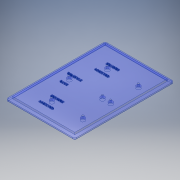
# Autodesk Inventor part: top
Saved by Autodesk Inventor 2017 SP1 (Build 210196100, 196)
## iProperties
Created: 2016-12-24
Part Number: top
Material: Generic
Document SubType Name: Modeling
Designer: wsh32
Density: 1 g/cm^3
Appearance: Clear - Blue
Author: wsh32
Autodesk Inventor part; units mm, degrees
(part 1 of 2)
ref_plane "YZ Plane" through (0, 0, 0) normal (1, 0, 0) x (0, 1, 0)
ref_plane "XZ Plane" through (0, 0, 0) normal (0, 1, 0) x (-1, 0, 0)
ref_plane "XY Plane" through (0, 0, 0) normal (0, 0, 1) x (1, 0, 0)
sketch "Sketch1" plane through (0, 0, 0) normal (0, 1, 0) x (-1, 0, 0)
  line L0 (0, 0) -> (-106.68, 0)
  line L1 (-106.68, 0) -> (-106.68, -153.67)
  line L2 (-106.68, -153.67) -> (0, -153.67)
  line L3 (0, -153.67) -> (0, 0)
  dimension "d0" = 153.67
  dimension "d1" = 106.68
  constraints: 8 end point, 2 parallel, 1 horizontal, 1 perpendicular
  measures "d0" distance of L2.end L0.start
  measures "d1" distance of L1.end L2.end
extrude "Extrusion1" add sketch "Sketch1" along normal blind 3.175
sketch "Sketch2" plane through (0, 3.175, 0) normal (0, 1, 0) x (1, 0, 0)
  line L0 (0, 0) -> (106.68, 0) projected
  line L1 (106.68, 0) -> (106.68, 153.67) projected
  line L2 (106.68, 153.67) -> (0, 153.67) projected
  line L3 (0, 153.67) -> (0, 0) projected
  line L4 (5.08, 5.08) -> (101.6, 5.08)
  line L5 (101.6, 5.08) -> (101.6, 148.59)
  line L6 (101.6, 148.59) -> (5.08, 148.59)
  line L7 (5.08, 148.59) -> (5.08, 5.08)
  dimension "d4" = 5.08
  constraints: 8 end point, 3 other
  measures "d4" distance between parallel lines of L3 L7
extrude "Extrusion2" add sketch "Sketch2" along normal blind 3.175 contours L7 L6 L5 L4
sketch "Sketch3" plane through (0, 0, 0) normal (0, -1, 0) x (1, 0, 0)
  line L0 (5.08, -5.08) -> (101.6, -5.08) construction
  line L1 (101.6, -5.08) -> (101.6, -148.59) construction
  line L2 (101.6, -148.59) -> (5.08, -148.59) construction
  line L3 (5.08, -148.59) -> (5.08, -5.08) construction
  line L4 (37.2533, -33.782) -> (85.5133, -33.782) construction
  line L5 (85.5133, -33.782) -> (85.5133, -119.888) construction
  line L6 (85.5133, -119.888) -> (37.2533, -119.888) construction
  line L7 (37.2533, -119.888) -> (37.2533, -33.782) construction
  line L8 (37.2533, -76.835) -> (85.5133, -76.835) construction
  point P0 (0, 0)
  point P1 (21.1667, -76.835)
  dimension "d7" = 28.702
  dimension "d8" = 28.702
  dimension "d9" = 16.0867
  dimension "d10" = 16.0867
  dimension "d11" = 16.0867
  dimension "d12" = 48.26
  dimension "d13" = 86.106
  constraints: 10 end point, 4 coincident, 2 midpoint, 2 parallel, 1 horizontal, 1 perpendicular, 1 point on line
  measures "d7" distance between parallel lines of L0 L4
  measures "d8" distance between parallel lines of L2 L6
  measures "d9" distance from line of L3 point (21.167, -76.835)
  measures "d10" distance from line of L7 point (21.167, -76.835)
  measures "d11" distance between parallel lines of L1 L5
  measures "d12" distance of L4.start L4.end
  measures "d13" distance of L4.end L5.end
hole "Hole1" at (37.2533, 0, -33.782) at (85.5133, 0, -33.782) at (21.1667, 0, -76.835) at (37.2533, 0, -119.888) at (85.5133, 0, -119.888) direction (0, 1, 0) diameter 3.175 end through all counterbore diameter 6.35 counterbore depth 3.175
sketch "Sketch4" plane through (0, 0, 0) normal (0, -1, 0) x (1, 0, 0)
  line L0 (31.5383, -22.987) -> (42.9683, -22.987) construction
  line L1 (42.9683, -22.987) -> (42.9683, -28.067) construction
  line L2 (42.9683, -28.067) -> (31.5383, -28.067) construction
  line L3 (31.5383, -28.067) -> (31.5383, -22.987) construction
  line L4 (31.5383, -39.497) -> (42.9683, -39.497) construction
  line L5 (42.9683, -39.497) -> (42.9683, -44.577) construction
  line L6 (42.9683, -44.577) -> (31.5383, -44.577) construction
  line L7 (31.5383, -44.577) -> (31.5383, -39.497) construction
  line L8 (15.4517, -66.04) -> (26.8817, -66.04) construction
  line L9 (26.8817, -66.04) -> (26.8817, -71.12) construction
  line L10 (26.8817, -71.12) -> (15.4517, -71.12) construction
  line L11 (15.4517, -71.12) -> (15.4517, -66.04) construction
  line L12 (15.4517, -82.55) -> (26.8817, -82.55) construction
  line L13 (26.8817, -82.55) -> (26.8817, -87.63) construction
  line L14 (26.8817, -87.63) -> (15.4517, -87.63) construction
  line L15 (15.4517, -87.63) -> (15.4517, -82.55) construction
  line L16 (31.5383, -109.093) -> (42.9683, -109.093) construction
  line L17 (42.9683, -109.093) -> (42.9683, -114.173) construction
  line L18 (42.9683, -114.173) -> (31.5383, -114.173) construction
  line L19 (31.5383, -114.173) -> (31.5383, -109.093) construction
  line L20 (31.5383, -125.603) -> (42.9683, -125.603) construction
  line L21 (42.9683, -125.603) -> (42.9683, -130.683) construction
  line L22 (42.9683, -130.683) -> (31.5383, -130.683) construction
  line L23 (31.5383, -130.683) -> (31.5383, -125.603) construction
  circle A0 centre (37.2533, -119.888) radius 3.175 construction
  circle A1 centre (85.5133, -33.782) radius 3.175 construction
  circle A2 centre (37.2533, -33.782) radius 3.175 construction
  circle A3 centre (21.1667, -76.835) radius 3.175 construction
  circle A4 centre (85.5133, -119.888) radius 3.175 construction
  line L24 (0, 0) -> (106.68, 0) construction
  line L25 (0, -153.67) -> (0, 0) construction
  line L26 (106.68, -153.67) -> (0, -153.67) construction
  line L27 (106.68, 0) -> (106.68, -153.67) construction
  circle A5 centre (37.2533, -119.888) radius 5.715 construction
  circle A6 centre (21.1667, -76.835) radius 5.715 construction
  circle A7 centre (37.2533, -33.782) radius 5.715 construction
  line L28 (28.5589, -24.5835) -> (27.2794, -24.5835)
  line L29 (27.2794, -24.5835) -> (27.2794, -25.159)
  line L30 (27.2794, -25.159) -> (28.4576, -25.159)
  line L31 (28.4576, -25.159) -> (28.4576, -25.7394)
  line L32 (28.4576, -25.7394) -> (27.2794, -25.7394)
  line L33 (27.2794, -25.7394) -> (27.2794, -27.051)
  line L34 (27.2794, -27.051) -> (26.5186, -27.051)
  line L35 (26.5186, -27.051) -> (26.5186, -24.003)
  line L36 (26.5186, -24.003) -> (28.5589, -24.003)
  line L37 (28.5589, -24.003) -> (28.5589, -24.5835)
  spline S0 degree 2 poles (31.7279, -25.527) (31.7279, -26.268) (30.9375, -27.1152) (30.2508, -27.1152) knots 0 0 0 1 2 2 2
  spline S1 degree 2 poles (30.2508, -27.1152) (29.5617, -27.1152) (28.7762, -26.2581) (28.7762, -25.527) knots 0 0 0 1 2 2 2
  spline S2 degree 2 poles (28.7762, -25.527) (28.7762, -24.7934) (29.5617, -23.9388) (30.2508, -23.9388) knots 0 0 0 1 2 2 2
  spline S3 degree 2 poles (30.2508, -23.9388) (30.9375, -23.9388) (31.7279, -24.7885) (31.7279, -25.527) knots 0 0 0 1 2 2 2
  spline S4 degree 2 poles (30.9375, -25.527) (30.9375, -25.2528) (30.8264, -24.87) (30.73, -24.7489) knots 0 0 0 1 2 2 2
  spline S5 degree 2 poles (30.73, -24.7489) (30.6337, -24.623) (30.3867, -24.5143) (30.2533, -24.5143) knots 0 0 0 1 2 2 2
  spline S6 degree 2 poles (30.2533, -24.5143) (30.1125, -24.5143) (29.8828, -24.6156) (29.7766, -24.744) knots 0 0 0 1 2 2 2
  spline S7 degree 2 poles (29.7766, -24.744) (29.6827, -24.8626) (29.5666, -25.2553) (29.5666, -25.527) knots 0 0 0 1 2 2 2
  spline S8 degree 2 poles (29.5666, -25.527) (29.5666, -25.8086) (29.6778, -26.1791) (29.7741, -26.3051) knots 0 0 0 1 2 2 2
  spline S9 degree 2 poles (29.7741, -26.3051) (29.8705, -26.431) (30.1199, -26.5397) (30.2533, -26.5397) knots 0 0 0 1 2 2 2
  spline S10 degree 2 poles (30.2533, -26.5397) (30.3892, -26.5397) (30.6411, -26.4236) (30.7325, -26.3001) knots 0 0 0 1 2 2 2
  spline S11 degree 2 poles (30.7325, -26.3001) (30.8313, -26.1667) (30.9375, -25.8135) (30.9375, -25.527) knots 0 0 0 1 2 2 2
  line L38 (34.9982, -27.051) -> (34.067, -27.051)
  line L39 (34.067, -27.051) -> (33.2198, -25.9321)
  line L40 (33.2198, -25.9321) -> (32.9432, -25.9321)
  line L41 (32.9432, -25.9321) -> (32.9432, -27.051)
  line L42 (32.9432, -27.051) -> (32.1824, -27.051)
  line L43 (32.1824, -27.051) -> (32.1824, -24.003)
  line L44 (32.1824, -24.003) -> (33.4075, -24.003)
  spline S12 degree 2 poles (33.4075, -24.003) (33.6619, -24.003) (34.0374, -24.0672) (34.1979, -24.166) knots 0 0 0 1 2 2 2
  spline S13 degree 2 poles (34.1979, -24.166) (34.3609, -24.2698) (34.5536, -24.5933) (34.5536, -24.8403) knots 0 0 0 1 2 2 2
  spline S14 degree 2 poles (34.5536, -24.8403) (34.5536, -25.1886) (34.2374, -25.6258) (33.9732, -25.7542) knots 0 0 0 1 2 2 2
  line L45 (33.9732, -25.7542) -> (34.9982, -27.051)
  spline S15 degree 2 poles (33.7681, -24.9367) (33.7681, -24.8206) (33.6792, -24.6551) (33.5779, -24.6106) knots 0 0 0 1 2 2 2
  spline S16 degree 2 poles (33.5779, -24.6106) (33.5063, -24.581) (33.3309, -24.5637) (33.2, -24.5637) knots 0 0 0 1 2 2 2
  line L46 (33.2, -24.5637) -> (32.9432, -24.5637)
  line L47 (32.9432, -24.5637) -> (32.9432, -25.3837)
  line L48 (32.9432, -25.3837) -> (33.163, -25.3837)
  spline S17 degree 2 poles (33.163, -25.3837) (33.3211, -25.3837) (33.5458, -25.3442) (33.6224, -25.2825) knots 0 0 0 1 2 2 2
  spline S18 degree 2 poles (33.6224, -25.2825) (33.6965, -25.2232) (33.7681, -25.0651) (33.7681, -24.9367) knots 0 0 0 1 2 2 2
  line L49 (39.1552, -24.003) -> (38.3846, -27.051)
  line L50 (38.3846, -27.051) -> (37.5448, -27.051)
  line L51 (37.5448, -27.051) -> (37.0557, -25.1664)
  line L52 (37.0557, -25.1664) -> (36.584, -27.051)
  line L53 (36.584, -27.051) -> (35.7417, -27.051)
  line L54 (35.7417, -27.051) -> (34.971, -24.003)
  line L55 (34.971, -24.003) -> (35.7664, -24.003)
  line L56 (35.7664, -24.003) -> (36.1863, -26.0432)
  line L57 (36.1863, -26.0432) -> (36.6951, -24.003)
  line L58 (36.6951, -24.003) -> (37.4559, -24.003)
  line L59 (37.4559, -24.003) -> (37.94, -26.0457)
  line L60 (37.94, -26.0457) -> (38.3797, -24.003)
  line L61 (38.3797, -24.003) -> (39.1552, -24.003)
  line L62 (39.2046, -27.051) -> (40.2346, -24.003)
  line L63 (40.2346, -24.003) -> (41.0695, -24.003)
  line L64 (41.0695, -24.003) -> (42.0995, -27.051)
  line L65 (42.0995, -27.051) -> (41.3116, -27.051)
  line L66 (41.3116, -27.051) -> (41.1214, -26.4286)
  line L67 (41.1214, -26.4286) -> (40.163, -26.4286)
  line L68 (40.163, -26.4286) -> (39.9704, -27.051)
  line L69 (39.9704, -27.051) -> (39.2046, -27.051)
  line L70 (40.9534, -25.8753) -> (40.6422, -24.8675)
  line L71 (40.6422, -24.8675) -> (40.3285, -25.8753)
  line L72 (40.3285, -25.8753) -> (40.9534, -25.8753)
  line L73 (45.2191, -27.051) -> (44.2879, -27.051)
  line L74 (44.2879, -27.051) -> (43.4407, -25.9321)
  line L75 (43.4407, -25.9321) -> (43.1641, -25.9321)
  line L76 (43.1641, -25.9321) -> (43.1641, -27.051)
  line L77 (43.1641, -27.051) -> (42.4033, -27.051)
  line L78 (42.4033, -27.051) -> (42.4033, -24.003)
  line L79 (42.4033, -24.003) -> (43.6284, -24.003)
  spline S19 degree 2 poles (43.6284, -24.003) (43.8829, -24.003) (44.2583, -24.0672) (44.4189, -24.166) knots 0 0 0 1 2 2 2
  spline S20 degree 2 poles (44.4189, -24.166) (44.5819, -24.2698) (44.7745, -24.5933) (44.7745, -24.8403) knots 0 0 0 1 2 2 2
  spline S21 degree 2 poles (44.7745, -24.8403) (44.7745, -25.1886) (44.4584, -25.6258) (44.1941, -25.7542) knots 0 0 0 1 2 2 2
  line L80 (44.1941, -25.7542) -> (45.2191, -27.051)
  spline S22 degree 2 poles (43.9891, -24.9367) (43.9891, -24.8206) (43.9001, -24.6551) (43.7989, -24.6106) knots 0 0 0 1 2 2 2
  spline S23 degree 2 poles (43.7989, -24.6106) (43.7272, -24.581) (43.5519, -24.5637) (43.421, -24.5637) knots 0 0 0 1 2 2 2
  line L81 (43.421, -24.5637) -> (43.1641, -24.5637)
  line L82 (43.1641, -24.5637) -> (43.1641, -25.3837)
  line L83 (43.1641, -25.3837) -> (43.3839, -25.3837)
  spline S24 degree 2 poles (43.3839, -25.3837) (43.542, -25.3837) (43.7668, -25.3442) (43.8433, -25.2825) knots 0 0 0 1 2 2 2
  spline S25 degree 2 poles (43.8433, -25.2825) (43.9174, -25.2232) (43.9891, -25.0651) (43.9891, -24.9367) knots 0 0 0 1 2 2 2
  spline S26 degree 2 poles (48.1659, -25.5295) (48.1659, -25.9568) (47.7929, -26.6286) (47.5088, -26.8089) knots 0 0 0 1 2 2 2
  spline S27 degree 2 poles (47.5088, -26.8089) (47.2717, -26.9621) (46.7135, -27.051) (46.3998, -27.051) knots 0 0 0 1 2 2 2
  line L84 (46.3998, -27.051) -> (45.4464, -27.051)
  line L85 (45.4464, -27.051) -> (45.4464, -24.003)
  line L86 (45.4464, -24.003) -> (46.3899, -24.003)
  spline S28 degree 2 poles (46.3899, -24.003) (46.711, -24.003) (47.2717, -24.0845) (47.5187, -24.2426) knots 0 0 0 1 2 2 2
  spline S29 degree 2 poles (47.5187, -24.2426) (47.8176, -24.4353) (48.1659, -25.0873) (48.1659, -25.5295) knots 0 0 0 1 2 2 2
  spline S30 degree 2 poles (47.3804, -25.5245) (47.3804, -25.2232) (47.1729, -24.7934) (46.9605, -24.6724) knots 0 0 0 1 2 2 2
  spline S31 degree 2 poles (46.9605, -24.6724) (46.8049, -24.5884) (46.464, -24.5711) (46.2269, -24.5711) knots 0 0 0 1 2 2 2
  line L87 (46.2269, -24.5711) -> (46.2121, -24.5711)
  line L88 (46.2121, -24.5711) -> (46.2121, -26.4804)
  line L89 (46.2121, -26.4804) -> (46.2269, -26.4804)
  spline S32 degree 2 poles (46.2269, -26.4804) (46.4838, -26.4804) (46.837, -26.4631) (46.9975, -26.3619) knots 0 0 0 1 2 2 2
  spline S33 degree 2 poles (46.9975, -26.3619) (47.1853, -26.2433) (47.3804, -25.8259) (47.3804, -25.5245) knots 0 0 0 1 2 2 2
  line L90 (30.7325, -43.561) -> (29.8013, -43.561)
  line L91 (29.8013, -43.561) -> (28.9541, -42.4421)
  line L92 (28.9541, -42.4421) -> (28.6774, -42.4421)
  line L93 (28.6774, -42.4421) -> (28.6774, -43.561)
  line L94 (28.6774, -43.561) -> (27.9167, -43.561)
  line L95 (27.9167, -43.561) -> (27.9167, -40.513)
  line L96 (27.9167, -40.513) -> (29.1418, -40.513)
  spline S34 degree 2 poles (29.1418, -40.513) (29.3962, -40.513) (29.7717, -40.5772) (29.9322, -40.676) knots 0 0 0 1 2 2 2
  spline S35 degree 2 poles (29.9322, -40.676) (30.0952, -40.7798) (30.2879, -41.1033) (30.2879, -41.3503) knots 0 0 0 1 2 2 2
  spline S36 degree 2 poles (30.2879, -41.3503) (30.2879, -41.6986) (29.9717, -42.1358) (29.7074, -42.2642) knots 0 0 0 1 2 2 2
  line L97 (29.7074, -42.2642) -> (30.7325, -43.561)
  spline S37 degree 2 poles (29.5024, -41.4467) (29.5024, -41.3306) (29.4135, -41.1651) (29.3122, -41.1206) knots 0 0 0 1 2 2 2
  spline S38 degree 2 poles (29.3122, -41.1206) (29.2406, -41.091) (29.0652, -41.0737) (28.9343, -41.0737) knots 0 0 0 1 2 2 2
  line L98 (28.9343, -41.0737) -> (28.6774, -41.0737)
  line L99 (28.6774, -41.0737) -> (28.6774, -41.8937)
  line L100 (28.6774, -41.8937) -> (28.8973, -41.8937)
  spline S39 degree 2 poles (28.8973, -41.8937) (29.0553, -41.8937) (29.2801, -41.8542) (29.3567, -41.7925) knots 0 0 0 1 2 2 2
  spline S40 degree 2 poles (29.3567, -41.7925) (29.4308, -41.7332) (29.5024, -41.5751) (29.5024, -41.4467) knots 0 0 0 1 2 2 2
  line L101 (30.9597, -43.561) -> (30.9597, -40.513)
  line L102 (30.9597, -40.513) -> (33.0197, -40.513)
  line L103 (33.0197, -40.513) -> (33.0197, -41.0935)
  line L104 (33.0197, -41.0935) -> (31.7205, -41.0935)
  line L105 (31.7205, -41.0935) -> (31.7205, -41.6294)
  line L106 (31.7205, -41.6294) -> (32.9185, -41.6294)
  line L107 (32.9185, -41.6294) -> (32.9185, -42.2099)
  line L108 (32.9185, -42.2099) -> (31.7205, -42.2099)
  line L109 (31.7205, -42.2099) -> (31.7205, -42.9805)
  line L110 (31.7205, -42.9805) -> (33.0197, -42.9805)
  line L111 (33.0197, -42.9805) -> (33.0197, -43.561)
  line L112 (33.0197, -43.561) -> (30.9597, -43.561)
  line L113 (36.0825, -40.513) -> (35.0353, -43.561)
  line L114 (35.0353, -43.561) -> (34.2374, -43.561)
  line L115 (34.2374, -43.561) -> (33.1902, -40.513)
  line L116 (33.1902, -40.513) -> (33.983, -40.513)
  line L117 (33.983, -40.513) -> (34.6475, -42.5804)
  line L118 (34.6475, -42.5804) -> (35.3094, -40.513)
  line L119 (35.3094, -40.513) -> (36.0825, -40.513)
  line L120 (36.3666, -43.561) -> (36.3666, -40.513)
  line L121 (36.3666, -40.513) -> (38.4266, -40.513)
  line L122 (38.4266, -40.513) -> (38.4266, -41.0935)
  line L123 (38.4266, -41.0935) -> (37.1274, -41.0935)
  line L124 (37.1274, -41.0935) -> (37.1274, -41.6294)
  line L125 (37.1274, -41.6294) -> (38.3253, -41.6294)
  line L126 (38.3253, -41.6294) -> (38.3253, -42.2099)
  line L127 (38.3253, -42.2099) -> (37.1274, -42.2099)
  line L128 (37.1274, -42.2099) -> (37.1274, -42.9805)
  line L129 (37.1274, -42.9805) -> (38.4266, -42.9805)
  line L130 (38.4266, -42.9805) -> (38.4266, -43.561)
  line L131 (38.4266, -43.561) -> (36.3666, -43.561)
  line L132 (41.7611, -43.561) -> (40.8299, -43.561)
  line L133 (40.8299, -43.561) -> (39.9827, -42.4421)
  line L134 (39.9827, -42.4421) -> (39.7061, -42.4421)
  line L135 (39.7061, -42.4421) -> (39.7061, -43.561)
  line L136 (39.7061, -43.561) -> (38.9453, -43.561)
  line L137 (38.9453, -43.561) -> (38.9453, -40.513)
  line L138 (38.9453, -40.513) -> (40.1704, -40.513)
  spline S41 degree 2 poles (40.1704, -40.513) (40.4248, -40.513) (40.8003, -40.5772) (40.9608, -40.676) knots 0 0 0 1 2 2 2
  spline S42 degree 2 poles (40.9608, -40.676) (41.1238, -40.7798) (41.3165, -41.1033) (41.3165, -41.3503) knots 0 0 0 1 2 2 2
  spline S43 degree 2 poles (41.3165, -41.3503) (41.3165, -41.6986) (41.0003, -42.1358) (40.7361, -42.2642) knots 0 0 0 1 2 2 2
  line L139 (40.7361, -42.2642) -> (41.7611, -43.561)
  spline S44 degree 2 poles (40.531, -41.4467) (40.531, -41.3306) (40.4421, -41.1651) (40.3409, -41.1206) knots 0 0 0 1 2 2 2
  spline S45 degree 2 poles (40.3409, -41.1206) (40.2692, -41.091) (40.0939, -41.0737) (39.9629, -41.0737) knots 0 0 0 1 2 2 2
  line L140 (39.9629, -41.0737) -> (39.7061, -41.0737)
  line L141 (39.7061, -41.0737) -> (39.7061, -41.8937)
  line L142 (39.7061, -41.8937) -> (39.9259, -41.8937)
  spline S46 degree 2 poles (39.9259, -41.8937) (40.084, -41.8937) (40.3087, -41.8542) (40.3853, -41.7925) knots 0 0 0 1 2 2 2
  spline S47 degree 2 poles (40.3853, -41.7925) (40.4594, -41.7332) (40.531, -41.5751) (40.531, -41.4467) knots 0 0 0 1 2 2 2
  spline S48 degree 2 poles (42.9294, -43.6153) (42.5787, -43.6153) (42.0501, -43.4795) (41.8229, -43.3807) knots 0 0 0 1 2 2 2
  line L143 (41.8229, -43.3807) -> (41.8229, -42.6545)
  line L144 (41.8229, -42.6545) -> (41.892, -42.6545)
  spline S49 degree 2 poles (41.892, -42.6545) (42.1217, -42.8496) (42.6725, -43.0596) (42.9319, -43.0596) knots 0 0 0 1 2 2 2
  spline S50 degree 2 poles (42.9319, -43.0596) (42.9986, -43.0596) (43.2135, -43.0299) (43.2777, -43.0003) knots 0 0 0 1 2 2 2
  spline S51 degree 2 poles (43.2777, -43.0003) (43.3567, -42.9657) (43.4679, -42.8398) (43.4679, -42.7385) knots 0 0 0 1 2 2 2
  spline S52 degree 2 poles (43.4679, -42.7385) (43.4679, -42.6224) (43.2876, -42.4791) (43.1641, -42.447) knots 0 0 0 1 2 2 2
  spline S53 degree 2 poles (43.1641, -42.447) (43.0085, -42.405) (42.6553, -42.3334) (42.4996, -42.2791) knots 0 0 0 1 2 2 2
  spline S54 degree 2 poles (42.4996, -42.2791) (42.1464, -42.1556) (41.8402, -41.7332) (41.8402, -41.417) knots 0 0 0 1 2 2 2
  spline S55 degree 2 poles (41.8402, -41.417) (41.8402, -40.9897) (42.5639, -40.4587) (43.1073, -40.4587) knots 0 0 0 1 2 2 2
  spline S56 degree 2 poles (43.1073, -40.4587) (43.379, -40.4587) (43.9174, -40.5698) (44.1299, -40.6637) knots 0 0 0 1 2 2 2
  line L145 (44.1299, -40.6637) -> (44.1299, -41.3602)
  line L146 (44.1299, -41.3602) -> (44.0632, -41.3602)
  spline S57 degree 2 poles (44.0632, -41.3602) (43.8927, -41.2145) (43.4037, -41.0144) (43.1468, -41.0144) knots 0 0 0 1 2 2 2
  spline S58 degree 2 poles (43.1468, -41.0144) (43.0455, -41.0144) (42.8874, -41.0441) (42.7985, -41.0836) knots 0 0 0 1 2 2 2
  spline S59 degree 2 poles (42.7985, -41.0836) (42.7269, -41.1157) (42.6231, -41.2441) (42.6231, -41.3232) knots 0 0 0 1 2 2 2
  spline S60 degree 2 poles (42.6231, -41.3232) (42.6231, -41.4417) (42.7886, -41.5776) (43.0258, -41.6319) knots 0 0 0 1 2 2 2
  spline S61 degree 2 poles (43.0258, -41.6319) (43.1789, -41.6665) (43.463, -41.7332) (43.626, -41.79) knots 0 0 0 1 2 2 2
  spline S62 degree 2 poles (43.626, -41.79) (43.9421, -41.9061) (44.2509, -42.2914) (44.2509, -42.6076) knots 0 0 0 1 2 2 2
  spline S63 degree 2 poles (44.2509, -42.6076) (44.2509, -43.0621) (43.5371, -43.6153) (42.9294, -43.6153) knots 0 0 0 1 2 2 2
  line L147 (44.6436, -43.561) -> (44.6436, -40.513)
  line L148 (44.6436, -40.513) -> (46.7036, -40.513)
  line L149 (46.7036, -40.513) -> (46.7036, -41.0935)
  line L150 (46.7036, -41.0935) -> (45.4044, -41.0935)
  line L151 (45.4044, -41.0935) -> (45.4044, -41.6294)
  line L152 (45.4044, -41.6294) -> (46.6023, -41.6294)
  line L153 (46.6023, -41.6294) -> (46.6023, -42.2099)
  line L154 (46.6023, -42.2099) -> (45.4044, -42.2099)
  line L155 (45.4044, -42.2099) -> (45.4044, -42.9805)
  line L156 (45.4044, -42.9805) -> (46.7036, -42.9805)
  line L157 (46.7036, -42.9805) -> (46.7036, -43.561)
  line L158 (46.7036, -43.561) -> (44.6436, -43.561)
  spline S64 degree 2 poles (16.6762, -70.1583) (16.3254, -70.1583) (15.7969, -70.0225) (15.5696, -69.9237) knots 0 0 0 1 2 2 2
  line L159 (15.5696, -69.9237) -> (15.5696, -69.1975)
  line L160 (15.5696, -69.1975) -> (15.6388, -69.1975)
  spline S65 degree 2 poles (15.6388, -69.1975) (15.8685, -69.3926) (16.4193, -69.6026) (16.6786, -69.6026) knots 0 0 0 1 2 2 2
  spline S66 degree 2 poles (16.6786, -69.6026) (16.7453, -69.6026) (16.9602, -69.5729) (17.0244, -69.5433) knots 0 0 0 1 2 2 2
  spline S67 degree 2 poles (17.0244, -69.5433) (17.1035, -69.5087) (17.2146, -69.3828) (17.2146, -69.2815) knots 0 0 0 1 2 2 2
  spline S68 degree 2 poles (17.2146, -69.2815) (17.2146, -69.1654) (17.0343, -69.0221) (16.9108, -68.99) knots 0 0 0 1 2 2 2
  spline S69 degree 2 poles (16.9108, -68.99) (16.7552, -68.948) (16.402, -68.8764) (16.2464, -68.8221) knots 0 0 0 1 2 2 2
  spline S70 degree 2 poles (16.2464, -68.8221) (15.8932, -68.6986) (15.5869, -68.2762) (15.5869, -67.96) knots 0 0 0 1 2 2 2
  spline S71 degree 2 poles (15.5869, -67.96) (15.5869, -67.5327) (16.3106, -67.0017) (16.854, -67.0017) knots 0 0 0 1 2 2 2
  spline S72 degree 2 poles (16.854, -67.0017) (17.1257, -67.0017) (17.6642, -67.1128) (17.8766, -67.2067) knots 0 0 0 1 2 2 2
  line L161 (17.8766, -67.2067) -> (17.8766, -67.9032)
  line L162 (17.8766, -67.9032) -> (17.8099, -67.9032)
  spline S73 degree 2 poles (17.8099, -67.9032) (17.6395, -67.7575) (17.1504, -67.5574) (16.8935, -67.5574) knots 0 0 0 1 2 2 2
  spline S74 degree 2 poles (16.8935, -67.5574) (16.7923, -67.5574) (16.6342, -67.5871) (16.5453, -67.6266) knots 0 0 0 1 2 2 2
  spline S75 degree 2 poles (16.5453, -67.6266) (16.4736, -67.6587) (16.3699, -67.7871) (16.3699, -67.8662) knots 0 0 0 1 2 2 2
  spline S76 degree 2 poles (16.3699, -67.8662) (16.3699, -67.9847) (16.5354, -68.1206) (16.7725, -68.1749) knots 0 0 0 1 2 2 2
  spline S77 degree 2 poles (16.7725, -68.1749) (16.9256, -68.2095) (17.2097, -68.2762) (17.3727, -68.333) knots 0 0 0 1 2 2 2
  spline S78 degree 2 poles (17.3727, -68.333) (17.6889, -68.4491) (17.9976, -68.8344) (17.9976, -69.1506) knots 0 0 0 1 2 2 2
  spline S79 degree 2 poles (17.9976, -69.1506) (17.9976, -69.6051) (17.2838, -70.1583) (16.6762, -70.1583) knots 0 0 0 1 2 2 2
  line L163 (20.9246, -67.056) -> (19.8724, -68.8319)
  line L164 (19.8724, -68.8319) -> (19.8724, -70.104)
  line L165 (19.8724, -70.104) -> (19.1067, -70.104)
  line L166 (19.1067, -70.104) -> (19.1067, -68.869)
  line L167 (19.1067, -68.869) -> (18.0372, -67.056)
  line L168 (18.0372, -67.056) -> (18.9091, -67.056)
  line L169 (18.9091, -67.056) -> (19.5043, -68.1428)
  line L170 (19.5043, -68.1428) -> (20.0799, -67.056)
  line L171 (20.0799, -67.056) -> (20.9246, -67.056)
  line L172 (23.8121, -70.104) -> (23.076, -70.104)
  line L173 (23.076, -70.104) -> (21.9003, -67.9798)
  line L174 (21.9003, -67.9798) -> (21.9003, -70.104)
  line L175 (21.9003, -70.104) -> (21.2012, -70.104)
  line L176 (21.2012, -70.104) -> (21.2012, -67.056)
  line L177 (21.2012, -67.056) -> (22.1399, -67.056)
  line L178 (22.1399, -67.056) -> (23.113, -68.8023)
  line L179 (23.113, -68.8023) -> (23.113, -67.056)
  line L180 (23.113, -67.056) -> (23.8121, -67.056)
  line L181 (23.8121, -67.056) -> (23.8121, -70.104)
  spline S80 degree 2 poles (25.7461, -70.1633) (25.0594, -70.1633) (24.2542, -69.3334) (24.2542, -68.5825) knots 0 0 0 1 2 2 2
  spline S81 degree 2 poles (24.2542, -68.5825) (24.2542, -67.8588) (25.0619, -66.9967) (25.7485, -66.9967) knots 0 0 0 1 2 2 2
  spline S82 degree 2 poles (25.7485, -66.9967) (25.9289, -66.9967) (26.2203, -67.0387) (26.3537, -67.0733) knots 0 0 0 1 2 2 2
  spline S83 degree 2 poles (26.3537, -67.0733) (26.4574, -67.1054) (26.702, -67.2116) (26.7785, -67.2511) knots 0 0 0 1 2 2 2
  line L182 (26.7785, -67.2511) -> (26.7785, -67.9773)
  line L183 (26.7785, -67.9773) -> (26.702, -67.9773)
  spline S84 degree 2 poles (26.702, -67.9773) (26.6452, -67.9279) (26.4772, -67.7896) (26.371, -67.7254) knots 0 0 0 1 2 2 2
  spline S85 degree 2 poles (26.371, -67.7254) (26.2648, -67.6587) (26.0104, -67.5673) (25.8696, -67.5673) knots 0 0 0 1 2 2 2
  spline S86 degree 2 poles (25.8696, -67.5673) (25.7041, -67.5673) (25.4299, -67.671) (25.3039, -67.8019) knots 0 0 0 1 2 2 2
  spline S87 degree 2 poles (25.3039, -67.8019) (25.1903, -67.918) (25.0446, -68.3157) (25.0446, -68.5849) knots 0 0 0 1 2 2 2
  spline S88 degree 2 poles (25.0446, -68.5849) (25.0446, -68.869) (25.1953, -69.2568) (25.3188, -69.3753) knots 0 0 0 1 2 2 2
  spline S89 degree 2 poles (25.3188, -69.3753) (25.4373, -69.4914) (25.7288, -69.5927) (25.8745, -69.5927) knots 0 0 0 1 2 2 2
  spline S90 degree 2 poles (25.8745, -69.5927) (26.0252, -69.5927) (26.2994, -69.4914) (26.3932, -69.4297) knots 0 0 0 1 2 2 2
  spline S91 degree 2 poles (26.3932, -69.4297) (26.497, -69.3679) (26.6526, -69.237) (26.7094, -69.1852) knots 0 0 0 1 2 2 2
  line L184 (26.7094, -69.1852) -> (26.7785, -69.1852)
  line L185 (26.7785, -69.1852) -> (26.7785, -69.9015)
  spline S92 degree 2 poles (26.7785, -69.9015) (26.6946, -69.941) (26.4747, -70.0398) (26.3562, -70.0744) knots 0 0 0 1 2 2 2
  spline S93 degree 2 poles (26.3562, -70.0744) (26.2129, -70.1188) (25.9634, -70.1633) (25.7461, -70.1633) knots 0 0 0 1 2 2 2
  spline S94 degree 2 poles (11.6114, -86.6683) (11.2607, -86.6683) (10.7321, -86.5325) (10.5048, -86.4337) knots 0 0 0 1 2 2 2
  line L186 (10.5048, -86.4337) -> (10.5048, -85.7075)
  line L187 (10.5048, -85.7075) -> (10.574, -85.7075)
  spline S95 degree 2 poles (10.574, -85.7075) (10.8037, -85.9026) (11.3545, -86.1126) (11.6139, -86.1126) knots 0 0 0 1 2 2 2
  spline S96 degree 2 poles (11.6139, -86.1126) (11.6806, -86.1126) (11.8955, -86.0829) (11.9597, -86.0533) knots 0 0 0 1 2 2 2
  spline S97 degree 2 poles (11.9597, -86.0533) (12.0387, -86.0187) (12.1499, -85.8928) (12.1499, -85.7915) knots 0 0 0 1 2 2 2
  spline S98 degree 2 poles (12.1499, -85.7915) (12.1499, -85.6754) (11.9696, -85.5321) (11.8461, -85.5) knots 0 0 0 1 2 2 2
  spline S99 degree 2 poles (11.8461, -85.5) (11.6904, -85.458) (11.3372, -85.3864) (11.1816, -85.3321) knots 0 0 0 1 2 2 2
  spline S100 degree 2 poles (11.1816, -85.3321) (10.8284, -85.2086) (10.5221, -84.7862) (10.5221, -84.47) knots 0 0 0 1 2 2 2
  spline S101 degree 2 poles (10.5221, -84.47) (10.5221, -84.0427) (11.2458, -83.5117) (11.7893, -83.5117) knots 0 0 0 1 2 2 2
  spline S102 degree 2 poles (11.7893, -83.5117) (12.061, -83.5117) (12.5994, -83.6228) (12.8118, -83.7167) knots 0 0 0 1 2 2 2
  line L188 (12.8118, -83.7167) -> (12.8118, -84.4132)
  line L189 (12.8118, -84.4132) -> (12.7451, -84.4132)
  spline S103 degree 2 poles (12.7451, -84.4132) (12.5747, -84.2675) (12.0857, -84.0674) (11.8288, -84.0674) knots 0 0 0 1 2 2 2
  spline S104 degree 2 poles (11.8288, -84.0674) (11.7275, -84.0674) (11.5694, -84.0971) (11.4805, -84.1366) knots 0 0 0 1 2 2 2
  spline S105 degree 2 poles (11.4805, -84.1366) (11.4089, -84.1687) (11.3051, -84.2971) (11.3051, -84.3762) knots 0 0 0 1 2 2 2
  spline S106 degree 2 poles (11.3051, -84.3762) (11.3051, -84.4947) (11.4706, -84.6306) (11.7077, -84.6849) knots 0 0 0 1 2 2 2
  spline S107 degree 2 poles (11.7077, -84.6849) (11.8609, -84.7195) (12.1449, -84.7862) (12.308, -84.843) knots 0 0 0 1 2 2 2
  spline S108 degree 2 poles (12.308, -84.843) (12.6241, -84.9591) (12.9329, -85.3444) (12.9329, -85.6606) knots 0 0 0 1 2 2 2
  spline S109 degree 2 poles (12.9329, -85.6606) (12.9329, -86.1151) (12.219, -86.6683) (11.6114, -86.6683) knots 0 0 0 1 2 2 2
  line L190 (13.3256, -86.614) -> (13.3256, -83.566)
  line L191 (13.3256, -83.566) -> (15.3856, -83.566)
  line L192 (15.3856, -83.566) -> (15.3856, -84.1465)
  line L193 (15.3856, -84.1465) -> (14.0864, -84.1465)
  line L194 (14.0864, -84.1465) -> (14.0864, -84.6824)
  line L195 (14.0864, -84.6824) -> (15.2843, -84.6824)
  line L196 (15.2843, -84.6824) -> (15.2843, -85.2629)
  line L197 (15.2843, -85.2629) -> (14.0864, -85.2629)
  line L198 (14.0864, -85.2629) -> (14.0864, -86.0335)
  line L199 (14.0864, -86.0335) -> (15.3856, -86.0335)
  line L200 (15.3856, -86.0335) -> (15.3856, -86.614)
  line L201 (15.3856, -86.614) -> (13.3256, -86.614)
  spline S110 degree 2 poles (18.2483, -84.5268) (18.2483, -84.7393) (18.1125, -85.1246) (17.9865, -85.253) knots 0 0 0 1 2 2 2
  spline S111 degree 2 poles (17.9865, -85.253) (17.91, -85.3345) (17.7222, -85.4679) (17.6111, -85.5148) knots 0 0 0 1 2 2 2
  spline S112 degree 2 poles (17.6111, -85.5148) (17.4975, -85.5618) (17.2332, -85.6161) (17.0701, -85.6161) knots 0 0 0 1 2 2 2
  line L202 (17.0701, -85.6161) -> (16.67, -85.6161)
  line L203 (16.67, -85.6161) -> (16.67, -86.614)
  line L204 (16.67, -86.614) -> (15.9043, -86.614)
  line L205 (15.9043, -86.614) -> (15.9043, -83.566)
  line L206 (15.9043, -83.566) -> (17.0874, -83.566)
  spline S113 degree 2 poles (17.0874, -83.566) (17.3493, -83.566) (17.7321, -83.6623) (17.8877, -83.7661) knots 0 0 0 1 2 2 2
  spline S114 degree 2 poles (17.8877, -83.7661) (18.0606, -83.8822) (18.2483, -84.2625) (18.2483, -84.5268) knots 0 0 0 1 2 2 2
  spline S115 degree 2 poles (17.4629, -84.5466) (17.4629, -84.4157) (17.3394, -84.2304) (17.2554, -84.1959) knots 0 0 0 1 2 2 2
  spline S116 degree 2 poles (17.2554, -84.1959) (17.1467, -84.1489) (16.9491, -84.1341) (16.7787, -84.1341) knots 0 0 0 1 2 2 2
  line L207 (16.7787, -84.1341) -> (16.67, -84.1341)
  line L208 (16.67, -84.1341) -> (16.67, -85.048)
  line L209 (16.67, -85.048) -> (16.7243, -85.048)
  spline S117 degree 2 poles (16.7243, -85.048) (16.8306, -85.048) (17.0232, -85.0431) (17.0948, -85.0307) knots 0 0 0 1 2 2 2
  spline S118 degree 2 poles (17.0948, -85.0307) (17.1566, -85.0208) (17.2924, -84.9616) (17.3295, -84.9245) knots 0 0 0 1 2 2 2
  spline S119 degree 2 poles (17.3295, -84.9245) (17.4085, -84.8504) (17.4629, -84.6849) (17.4629, -84.5466) knots 0 0 0 1 2 2 2
  line L210 (18.6584, -86.614) -> (18.6584, -83.566)
  line L211 (18.6584, -83.566) -> (20.7184, -83.566)
  line L212 (20.7184, -83.566) -> (20.7184, -84.1465)
  line L213 (20.7184, -84.1465) -> (19.4191, -84.1465)
  line L214 (19.4191, -84.1465) -> (19.4191, -84.6824)
  line L215 (19.4191, -84.6824) -> (20.6171, -84.6824)
  line L216 (20.6171, -84.6824) -> (20.6171, -85.2629)
  line L217 (20.6171, -85.2629) -> (19.4191, -85.2629)
  line L218 (19.4191, -85.2629) -> (19.4191, -86.0335)
  line L219 (19.4191, -86.0335) -> (20.7184, -86.0335)
  line L220 (20.7184, -86.0335) -> (20.7184, -86.614)
  line L221 (20.7184, -86.614) -> (18.6584, -86.614)
  line L222 (24.0529, -86.614) -> (23.1217, -86.614)
  line L223 (23.1217, -86.614) -> (22.2745, -85.4951)
  line L224 (22.2745, -85.4951) -> (21.9978, -85.4951)
  line L225 (21.9978, -85.4951) -> (21.9978, -86.614)
  line L226 (21.9978, -86.614) -> (21.2371, -86.614)
  line L227 (21.2371, -86.614) -> (21.2371, -83.566)
  line L228 (21.2371, -83.566) -> (22.4622, -83.566)
  spline S120 degree 2 poles (22.4622, -83.566) (22.7166, -83.566) (23.092, -83.6302) (23.2526, -83.729) knots 0 0 0 1 2 2 2
  spline S121 degree 2 poles (23.2526, -83.729) (23.4156, -83.8328) (23.6083, -84.1563) (23.6083, -84.4033) knots 0 0 0 1 2 2 2
  spline S122 degree 2 poles (23.6083, -84.4033) (23.6083, -84.7516) (23.2921, -85.1888) (23.0278, -85.3172) knots 0 0 0 1 2 2 2
  line L229 (23.0278, -85.3172) -> (24.0529, -86.614)
  spline S123 degree 2 poles (22.8228, -84.4997) (22.8228, -84.3836) (22.7339, -84.2181) (22.6326, -84.1736) knots 0 0 0 1 2 2 2
  spline S124 degree 2 poles (22.6326, -84.1736) (22.561, -84.144) (22.3856, -84.1267) (22.2547, -84.1267) knots 0 0 0 1 2 2 2
  line L230 (22.2547, -84.1267) -> (21.9978, -84.1267)
  line L231 (21.9978, -84.1267) -> (21.9978, -84.9467)
  line L232 (21.9978, -84.9467) -> (22.2177, -84.9467)
  spline S125 degree 2 poles (22.2177, -84.9467) (22.3757, -84.9467) (22.6005, -84.9072) (22.6771, -84.8455) knots 0 0 0 1 2 2 2
  spline S126 degree 2 poles (22.6771, -84.8455) (22.7512, -84.7862) (22.8228, -84.6281) (22.8228, -84.4997) knots 0 0 0 1 2 2 2
  line L233 (23.9516, -86.614) -> (24.9816, -83.566)
  line L234 (24.9816, -83.566) -> (25.8165, -83.566)
  line L235 (25.8165, -83.566) -> (26.8465, -86.614)
  line L236 (26.8465, -86.614) -> (26.0585, -86.614)
  line L237 (26.0585, -86.614) -> (25.8683, -85.9916)
  line L238 (25.8683, -85.9916) -> (24.91, -85.9916)
  line L239 (24.91, -85.9916) -> (24.7173, -86.614)
  line L240 (24.7173, -86.614) -> (23.9516, -86.614)
  line L241 (25.7004, -85.4383) -> (25.3892, -84.4305)
  line L242 (25.3892, -84.4305) -> (25.0755, -85.4383)
  line L243 (25.0755, -85.4383) -> (25.7004, -85.4383)
  line L244 (27.7357, -86.614) -> (27.7357, -84.1465)
  line L245 (27.7357, -84.1465) -> (26.8341, -84.1465)
  line L246 (26.8341, -84.1465) -> (26.8341, -83.566)
  line L247 (26.8341, -83.566) -> (29.4029, -83.566)
  line L248 (29.4029, -83.566) -> (29.4029, -84.1465)
  line L249 (29.4029, -84.1465) -> (28.5014, -84.1465)
  line L250 (28.5014, -84.1465) -> (28.5014, -86.614)
  line L251 (28.5014, -86.614) -> (27.7357, -86.614)
  line L252 (29.7166, -86.614) -> (29.7166, -83.566)
  line L253 (29.7166, -83.566) -> (31.7766, -83.566)
  line L254 (31.7766, -83.566) -> (31.7766, -84.1465)
  line L255 (31.7766, -84.1465) -> (30.4774, -84.1465)
  line L256 (30.4774, -84.1465) -> (30.4774, -84.6824)
  line L257 (30.4774, -84.6824) -> (31.6754, -84.6824)
  line L258 (31.6754, -84.6824) -> (31.6754, -85.2629)
  line L259 (31.6754, -85.2629) -> (30.4774, -85.2629)
  line L260 (30.4774, -85.2629) -> (30.4774, -86.0335)
  line L261 (30.4774, -86.0335) -> (31.7766, -86.0335)
  line L262 (31.7766, -86.0335) -> (31.7766, -86.614)
  line L263 (31.7766, -86.614) -> (29.7166, -86.614)
  line L264 (28.5589, -110.6895) -> (27.2794, -110.6895)
  line L265 (27.2794, -110.6895) -> (27.2794, -111.265)
  line L266 (27.2794, -111.265) -> (28.4576, -111.265)
  line L267 (28.4576, -111.265) -> (28.4576, -111.8454)
  line L268 (28.4576, -111.8454) -> (27.2794, -111.8454)
  line L269 (27.2794, -111.8454) -> (27.2794, -113.157)
  line L270 (27.2794, -113.157) -> (26.5186, -113.157)
  line L271 (26.5186, -113.157) -> (26.5186, -110.109)
  line L272 (26.5186, -110.109) -> (28.5589, -110.109)
  line L273 (28.5589, -110.109) -> (28.5589, -110.6895)
  spline S127 degree 2 poles (31.7279, -111.633) (31.7279, -112.374) (30.9375, -113.2212) (30.2508, -113.2212) knots 0 0 0 1 2 2 2
  spline S128 degree 2 poles (30.2508, -113.2212) (29.5617, -113.2212) (28.7762, -112.3641) (28.7762, -111.633) knots 0 0 0 1 2 2 2
  spline S129 degree 2 poles (28.7762, -111.633) (28.7762, -110.8994) (29.5617, -110.0448) (30.2508, -110.0448) knots 0 0 0 1 2 2 2
  spline S130 degree 2 poles (30.2508, -110.0448) (30.9375, -110.0448) (31.7279, -110.8945) (31.7279, -111.633) knots 0 0 0 1 2 2 2
  spline S131 degree 2 poles (30.9375, -111.633) (30.9375, -111.3588) (30.8264, -110.976) (30.73, -110.8549) knots 0 0 0 1 2 2 2
  spline S132 degree 2 poles (30.73, -110.8549) (30.6337, -110.729) (30.3867, -110.6203) (30.2533, -110.6203) knots 0 0 0 1 2 2 2
  spline S133 degree 2 poles (30.2533, -110.6203) (30.1125, -110.6203) (29.8828, -110.7216) (29.7766, -110.85) knots 0 0 0 1 2 2 2
  spline S134 degree 2 poles (29.7766, -110.85) (29.6827, -110.9686) (29.5666, -111.3613) (29.5666, -111.633) knots 0 0 0 1 2 2 2
  spline S135 degree 2 poles (29.5666, -111.633) (29.5666, -111.9146) (29.6778, -112.2851) (29.7741, -112.4111) knots 0 0 0 1 2 2 2
  spline S136 degree 2 poles (29.7741, -112.4111) (29.8705, -112.537) (30.1199, -112.6457) (30.2533, -112.6457) knots 0 0 0 1 2 2 2
  spline S137 degree 2 poles (30.2533, -112.6457) (30.3892, -112.6457) (30.6411, -112.5296) (30.7325, -112.4061) knots 0 0 0 1 2 2 2
  spline S138 degree 2 poles (30.7325, -112.4061) (30.8313, -112.2727) (30.9375, -111.9195) (30.9375, -111.633) knots 0 0 0 1 2 2 2
  line L274 (34.9982, -113.157) -> (34.067, -113.157)
  line L275 (34.067, -113.157) -> (33.2198, -112.0381)
  line L276 (33.2198, -112.0381) -> (32.9432, -112.0381)
  line L277 (32.9432, -112.0381) -> (32.9432, -113.157)
  line L278 (32.9432, -113.157) -> (32.1824, -113.157)
  line L279 (32.1824, -113.157) -> (32.1824, -110.109)
  line L280 (32.1824, -110.109) -> (33.4075, -110.109)
  spline S139 degree 2 poles (33.4075, -110.109) (33.6619, -110.109) (34.0374, -110.1732) (34.1979, -110.272) knots 0 0 0 1 2 2 2
  spline S140 degree 2 poles (34.1979, -110.272) (34.3609, -110.3758) (34.5536, -110.6993) (34.5536, -110.9463) knots 0 0 0 1 2 2 2
  spline S141 degree 2 poles (34.5536, -110.9463) (34.5536, -111.2946) (34.2374, -111.7318) (33.9732, -111.8602) knots 0 0 0 1 2 2 2
  line L281 (33.9732, -111.8602) -> (34.9982, -113.157)
  spline S142 degree 2 poles (33.7681, -111.0427) (33.7681, -110.9266) (33.6792, -110.7611) (33.5779, -110.7166) knots 0 0 0 1 2 2 2
  spline S143 degree 2 poles (33.5779, -110.7166) (33.5063, -110.687) (33.3309, -110.6697) (33.2, -110.6697) knots 0 0 0 1 2 2 2
  line L282 (33.2, -110.6697) -> (32.9432, -110.6697)
  line L283 (32.9432, -110.6697) -> (32.9432, -111.4897)
  line L284 (32.9432, -111.4897) -> (33.163, -111.4897)
  spline S144 degree 2 poles (33.163, -111.4897) (33.3211, -111.4897) (33.5458, -111.4502) (33.6224, -111.3885) knots 0 0 0 1 2 2 2
  spline S145 degree 2 poles (33.6224, -111.3885) (33.6965, -111.3292) (33.7681, -111.1711) (33.7681, -111.0427) knots 0 0 0 1 2 2 2
  line L285 (39.1552, -110.109) -> (38.3846, -113.157)
  line L286 (38.3846, -113.157) -> (37.5448, -113.157)
  line L287 (37.5448, -113.157) -> (37.0557, -111.2724)
  line L288 (37.0557, -111.2724) -> (36.584, -113.157)
  line L289 (36.584, -113.157) -> (35.7417, -113.157)
  line L290 (35.7417, -113.157) -> (34.971, -110.109)
  line L291 (34.971, -110.109) -> (35.7664, -110.109)
  line L292 (35.7664, -110.109) -> (36.1863, -112.1492)
  line L293 (36.1863, -112.1492) -> (36.6951, -110.109)
  line L294 (36.6951, -110.109) -> (37.4559, -110.109)
  line L295 (37.4559, -110.109) -> (37.94, -112.1517)
  line L296 (37.94, -112.1517) -> (38.3797, -110.109)
  line L297 (38.3797, -110.109) -> (39.1552, -110.109)
  line L298 (39.2046, -113.157) -> (40.2346, -110.109)
  line L299 (40.2346, -110.109) -> (41.0695, -110.109)
  line L300 (41.0695, -110.109) -> (42.0995, -113.157)
  line L301 (42.0995, -113.157) -> (41.3116, -113.157)
  line L302 (41.3116, -113.157) -> (41.1214, -112.5346)
  line L303 (41.1214, -112.5346) -> (40.163, -112.5346)
  line L304 (40.163, -112.5346) -> (39.9704, -113.157)
  line L305 (39.9704, -113.157) -> (39.2046, -113.157)
  line L306 (40.9534, -111.9813) -> (40.6422, -110.9735)
  line L307 (40.6422, -110.9735) -> (40.3285, -111.9813)
  line L308 (40.3285, -111.9813) -> (40.9534, -111.9813)
  line L309 (45.2191, -113.157) -> (44.2879, -113.157)
  line L310 (44.2879, -113.157) -> (43.4407, -112.0381)
  line L311 (43.4407, -112.0381) -> (43.1641, -112.0381)
  line L312 (43.1641, -112.0381) -> (43.1641, -113.157)
  line L313 (43.1641, -113.157) -> (42.4033, -113.157)
  line L314 (42.4033, -113.157) -> (42.4033, -110.109)
  line L315 (42.4033, -110.109) -> (43.6284, -110.109)
  spline S146 degree 2 poles (43.6284, -110.109) (43.8829, -110.109) (44.2583, -110.1732) (44.4189, -110.272) knots 0 0 0 1 2 2 2
  spline S147 degree 2 poles (44.4189, -110.272) (44.5819, -110.3758) (44.7745, -110.6993) (44.7745, -110.9463) knots 0 0 0 1 2 2 2
  spline S148 degree 2 poles (44.7745, -110.9463) (44.7745, -111.2946) (44.4584, -111.7318) (44.1941, -111.8602) knots 0 0 0 1 2 2 2
  line L316 (44.1941, -111.8602) -> (45.2191, -113.157)
  spline S149 degree 2 poles (43.9891, -111.0427) (43.9891, -110.9266) (43.9001, -110.7611) (43.7989, -110.7166) knots 0 0 0 1 2 2 2
  spline S150 degree 2 poles (43.7989, -110.7166) (43.7272, -110.687) (43.5519, -110.6697) (43.421, -110.6697) knots 0 0 0 1 2 2 2
  line L317 (43.421, -110.6697) -> (43.1641, -110.6697)
  line L318 (43.1641, -110.6697) -> (43.1641, -111.4897)
  line L319 (43.1641, -111.4897) -> (43.3839, -111.4897)
  spline S151 degree 2 poles (43.3839, -111.4897) (43.542, -111.4897) (43.7668, -111.4502) (43.8433, -111.3885) knots 0 0 0 1 2 2 2
  spline S152 degree 2 poles (43.8433, -111.3885) (43.9174, -111.3292) (43.9891, -111.1711) (43.9891, -111.0427) knots 0 0 0 1 2 2 2
  spline S153 degree 2 poles (48.1659, -111.6355) (48.1659, -112.0628) (47.7929, -112.7346) (47.5088, -112.9149) knots 0 0 0 1 2 2 2
  spline S154 degree 2 poles (47.5088, -112.9149) (47.2717, -113.0681) (46.7135, -113.157) (46.3998, -113.157) knots 0 0 0 1 2 2 2
  line L320 (46.3998, -113.157) -> (45.4464, -113.157)
  line L321 (45.4464, -113.157) -> (45.4464, -110.109)
  line L322 (45.4464, -110.109) -> (46.3899, -110.109)
  spline S155 degree 2 poles (46.3899, -110.109) (46.711, -110.109) (47.2717, -110.1905) (47.5187, -110.3486) knots 0 0 0 1 2 2 2
  spline S156 degree 2 poles (47.5187, -110.3486) (47.8176, -110.5413) (48.1659, -111.1933) (48.1659, -111.6355) knots 0 0 0 1 2 2 2
  spline S157 degree 2 poles (47.3804, -111.6305) (47.3804, -111.3292) (47.1729, -110.8994) (46.9605, -110.7784) knots 0 0 0 1 2 2 2
  spline S158 degree 2 poles (46.9605, -110.7784) (46.8049, -110.6944) (46.464, -110.6771) (46.2269, -110.6771) knots 0 0 0 1 2 2 2
  line L323 (46.2269, -110.6771) -> (46.2121, -110.6771)
  line L324 (46.2121, -110.6771) -> (46.2121, -112.5864)
  line L325 (46.2121, -112.5864) -> (46.2269, -112.5864)
  spline S159 degree 2 poles (46.2269, -112.5864) (46.4838, -112.5864) (46.837, -112.5691) (46.9975, -112.4679) knots 0 0 0 1 2 2 2
  spline S160 degree 2 poles (46.9975, -112.4679) (47.1853, -112.3493) (47.3804, -111.9319) (47.3804, -111.6305) knots 0 0 0 1 2 2 2
  line L326 (30.7325, -129.667) -> (29.8013, -129.667)
  line L327 (29.8013, -129.667) -> (28.9541, -128.5481)
  line L328 (28.9541, -128.5481) -> (28.6774, -128.5481)
  line L329 (28.6774, -128.5481) -> (28.6774, -129.667)
  line L330 (28.6774, -129.667) -> (27.9167, -129.667)
  line L331 (27.9167, -129.667) -> (27.9167, -126.619)
  line L332 (27.9167, -126.619) -> (29.1418, -126.619)
  spline S161 degree 2 poles (29.1418, -126.619) (29.3962, -126.619) (29.7717, -126.6832) (29.9322, -126.782) knots 0 0 0 1 2 2 2
  spline S162 degree 2 poles (29.9322, -126.782) (30.0952, -126.8858) (30.2879, -127.2093) (30.2879, -127.4563) knots 0 0 0 1 2 2 2
  spline S163 degree 2 poles (30.2879, -127.4563) (30.2879, -127.8046) (29.9717, -128.2418) (29.7074, -128.3702) knots 0 0 0 1 2 2 2
  line L333 (29.7074, -128.3702) -> (30.7325, -129.667)
  spline S164 degree 2 poles (29.5024, -127.5527) (29.5024, -127.4366) (29.4135, -127.2711) (29.3122, -127.2266) knots 0 0 0 1 2 2 2
  spline S165 degree 2 poles (29.3122, -127.2266) (29.2406, -127.197) (29.0652, -127.1797) (28.9343, -127.1797) knots 0 0 0 1 2 2 2
  line L334 (28.9343, -127.1797) -> (28.6774, -127.1797)
  line L335 (28.6774, -127.1797) -> (28.6774, -127.9997)
  line L336 (28.6774, -127.9997) -> (28.8973, -127.9997)
  spline S166 degree 2 poles (28.8973, -127.9997) (29.0553, -127.9997) (29.2801, -127.9602) (29.3567, -127.8985) knots 0 0 0 1 2 2 2
  spline S167 degree 2 poles (29.3567, -127.8985) (29.4308, -127.8392) (29.5024, -127.6811) (29.5024, -127.5527) knots 0 0 0 1 2 2 2
  line L337 (30.9597, -129.667) -> (30.9597, -126.619)
  line L338 (30.9597, -126.619) -> (33.0197, -126.619)
  line L339 (33.0197, -126.619) -> (33.0197, -127.1995)
  line L340 (33.0197, -127.1995) -> (31.7205, -127.1995)
  line L341 (31.7205, -127.1995) -> (31.7205, -127.7354)
  line L342 (31.7205, -127.7354) -> (32.9185, -127.7354)
  line L343 (32.9185, -127.7354) -> (32.9185, -128.3159)
  line L344 (32.9185, -128.3159) -> (31.7205, -128.3159)
  line L345 (31.7205, -128.3159) -> (31.7205, -129.0865)
  line L346 (31.7205, -129.0865) -> (33.0197, -129.0865)
  line L347 (33.0197, -129.0865) -> (33.0197, -129.667)
  line L348 (33.0197, -129.667) -> (30.9597, -129.667)
  line L349 (36.0825, -126.619) -> (35.0353, -129.667)
  line L350 (35.0353, -129.667) -> (34.2374, -129.667)
  line L351 (34.2374, -129.667) -> (33.1902, -126.619)
  line L352 (33.1902, -126.619) -> (33.983, -126.619)
  line L353 (33.983, -126.619) -> (34.6475, -128.6864)
  line L354 (34.6475, -128.6864) -> (35.3094, -126.619)
  line L355 (35.3094, -126.619) -> (36.0825, -126.619)
  line L356 (36.3666, -129.667) -> (36.3666, -126.619)
  line L357 (36.3666, -126.619) -> (38.4266, -126.619)
  line L358 (38.4266, -126.619) -> (38.4266, -127.1995)
  line L359 (38.4266, -127.1995) -> (37.1274, -127.1995)
  line L360 (37.1274, -127.1995) -> (37.1274, -127.7354)
  line L361 (37.1274, -127.7354) -> (38.3253, -127.7354)
  line L362 (38.3253, -127.7354) -> (38.3253, -128.3159)
  line L363 (38.3253, -128.3159) -> (37.1274, -128.3159)
  line L364 (37.1274, -128.3159) -> (37.1274, -129.0865)
  line L365 (37.1274, -129.0865) -> (38.4266, -129.0865)
  line L366 (38.4266, -129.0865) -> (38.4266, -129.667)
  line L367 (38.4266, -129.667) -> (36.3666, -129.667)
  line L368 (41.7611, -129.667) -> (40.8299, -129.667)
  line L369 (40.8299, -129.667) -> (39.9827, -128.5481)
  line L370 (39.9827, -128.5481) -> (39.7061, -128.5481)
  line L371 (39.7061, -128.5481) -> (39.7061, -129.667)
  line L372 (39.7061, -129.667) -> (38.9453, -129.667)
  line L373 (38.9453, -129.667) -> (38.9453, -126.619)
  line L374 (38.9453, -126.619) -> (40.1704, -126.619)
  spline S168 degree 2 poles (40.1704, -126.619) (40.4248, -126.619) (40.8003, -126.6832) (40.9608, -126.782) knots 0 0 0 1 2 2 2
  spline S169 degree 2 poles (40.9608, -126.782) (41.1238, -126.8858) (41.3165, -127.2093) (41.3165, -127.4563) knots 0 0 0 1 2 2 2
  spline S170 degree 2 poles (41.3165, -127.4563) (41.3165, -127.8046) (41.0003, -128.2418) (40.7361, -128.3702) knots 0 0 0 1 2 2 2
  line L375 (40.7361, -128.3702) -> (41.7611, -129.667)
  spline S171 degree 2 poles (40.531, -127.5527) (40.531, -127.4366) (40.4421, -127.2711) (40.3409, -127.2266) knots 0 0 0 1 2 2 2
  spline S172 degree 2 poles (40.3409, -127.2266) (40.2692, -127.197) (40.0939, -127.1797) (39.9629, -127.1797) knots 0 0 0 1 2 2 2
  line L376 (39.9629, -127.1797) -> (39.7061, -127.1797)
  line L377 (39.7061, -127.1797) -> (39.7061, -127.9997)
  line L378 (39.7061, -127.9997) -> (39.9259, -127.9997)
  spline S173 degree 2 poles (39.9259, -127.9997) (40.084, -127.9997) (40.3087, -127.9602) (40.3853, -127.8985) knots 0 0 0 1 2 2 2
  spline S174 degree 2 poles (40.3853, -127.8985) (40.4594, -127.8392) (40.531, -127.6811) (40.531, -127.5527) knots 0 0 0 1 2 2 2
  spline S175 degree 2 poles (42.9294, -129.7213) (42.5787, -129.7213) (42.0501, -129.5855) (41.8229, -129.4867) knots 0 0 0 1 2 2 2
  line L379 (41.8229, -129.4867) -> (41.8229, -128.7605)
  line L380 (41.8229, -128.7605) -> (41.892, -128.7605)
  spline S176 degree 2 poles (41.892, -128.7605) (42.1217, -128.9556) (42.6725, -129.1656) (42.9319, -129.1656) knots 0 0 0 1 2 2 2
  spline S177 degree 2 poles (42.9319, -129.1656) (42.9986, -129.1656) (43.2135, -129.1359) (43.2777, -129.1063) knots 0 0 0 1 2 2 2
  spline S178 degree 2 poles (43.2777, -129.1063) (43.3567, -129.0717) (43.4679, -128.9458) (43.4679, -128.8445) knots 0 0 0 1 2 2 2
  spline S179 degree 2 poles (43.4679, -128.8445) (43.4679, -128.7284) (43.2876, -128.5851) (43.1641, -128.553) knots 0 0 0 1 2 2 2
  spline S180 degree 2 poles (43.1641, -128.553) (43.0085, -128.511) (42.6553, -128.4394) (42.4996, -128.3851) knots 0 0 0 1 2 2 2
  spline S181 degree 2 poles (42.4996, -128.3851) (42.1464, -128.2616) (41.8402, -127.8392) (41.8402, -127.523) knots 0 0 0 1 2 2 2
  spline S182 degree 2 poles (41.8402, -127.523) (41.8402, -127.0957) (42.5639, -126.5647) (43.1073, -126.5647) knots 0 0 0 1 2 2 2
  spline S183 degree 2 poles (43.1073, -126.5647) (43.379, -126.5647) (43.9174, -126.6758) (44.1299, -126.7697) knots 0 0 0 1 2 2 2
  line L381 (44.1299, -126.7697) -> (44.1299, -127.4662)
  line L382 (44.1299, -127.4662) -> (44.0632, -127.4662)
  spline S184 degree 2 poles (44.0632, -127.4662) (43.8927, -127.3205) (43.4037, -127.1204) (43.1468, -127.1204) knots 0 0 0 1 2 2 2
  spline S185 degree 2 poles (43.1468, -127.1204) (43.0455, -127.1204) (42.8874, -127.1501) (42.7985, -127.1896) knots 0 0 0 1 2 2 2
  spline S186 degree 2 poles (42.7985, -127.1896) (42.7269, -127.2217) (42.6231, -127.3501) (42.6231, -127.4292) knots 0 0 0 1 2 2 2
  spline S187 degree 2 poles (42.6231, -127.4292) (42.6231, -127.5477) (42.7886, -127.6836) (43.0258, -127.7379) knots 0 0 0 1 2 2 2
  spline S188 degree 2 poles (43.0258, -127.7379) (43.1789, -127.7725) (43.463, -127.8392) (43.626, -127.896) knots 0 0 0 1 2 2 2
  spline S189 degree 2 poles (43.626, -127.896) (43.9421, -128.0121) (44.2509, -128.3974) (44.2509, -128.7136) knots 0 0 0 1 2 2 2
  spline S190 degree 2 poles (44.2509, -128.7136) (44.2509, -129.1681) (43.5371, -129.7213) (42.9294, -129.7213) knots 0 0 0 1 2 2 2
  line L383 (44.6436, -129.667) -> (44.6436, -126.619)
  line L384 (44.6436, -126.619) -> (46.7036, -126.619)
  line L385 (46.7036, -126.619) -> (46.7036, -127.1995)
  line L386 (46.7036, -127.1995) -> (45.4044, -127.1995)
  line L387 (45.4044, -127.1995) -> (45.4044, -127.7354)
  line L388 (45.4044, -127.7354) -> (46.6023, -127.7354)
  line L389 (46.6023, -127.7354) -> (46.6023, -128.3159)
  line L390 (46.6023, -128.3159) -> (45.4044, -128.3159)